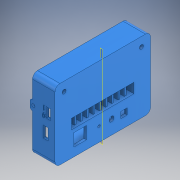
# Autodesk Inventor part: case_front
Saved by Autodesk Inventor 2018 (Build 220112000, 112)
## iProperties
Created: 2018-08-02
Part Number: case_front
Material: Generic
Document SubType Name: Modeling
Designer: Luke
Density: 1 g/cm^3
Appearance: Cyan
Author: Luke
Autodesk Inventor part; units mm, degrees
ref_plane "YZ Plane" through (0, 0, 0) normal (1, 0, 0) x (0, 1, 0)
ref_plane "XZ Plane" through (0, 0, 0) normal (0, 1, 0) x (-1, 0, 0)
sketch "Sketch1" plane through (0, 0, 0) normal (0, 1, 0) x (-1, 0, 0)
  line L0 (0, 0) -> (-76.5, 0)
  line L1 (-76.5, 0) -> (-76.5, 56.5)
  line L2 (-76.5, 56.5) -> (0, 56.5)
  line L3 (0, 56.5) -> (0, 0)
  dimension "d0" = 76.5
  dimension "d1" = 56.5
  constraints: 8 end point, 2 parallel, 1 horizontal, 1 perpendicular
  measures "d0" distance of L0.start L0.end
  measures "d1" distance of L0.end L1.end
extrude "Extrusion1" add sketch "Sketch1" along normal blind 2
ref_plane "Work Plane1" through (76.5, 0, 28.25) normal (0, 0, -1) x (-1, 0, 0)
ref_plane "Work Plane2" through (38.25, 0, 56.5) normal (1, 0, 0) x (0, 0, -1)
sketch "Sketch3" plane through (0, 2, 0) normal (0, 1, 0) x (1, 0, 0)
  line L0 (38.25, 11.3) -> (38.25, -67.8) construction
  line L1 (-15.3, -28.25) -> (91.8, -28.25) construction
  circle A0 centre (7.25, -7.25) radius 1.6
  circle A1 centre (69.25, -7.25) radius 1.6
  circle A2 centre (69.25, -49.25) radius 1.6
  circle A3 centre (7.25, -49.25) radius 1.6
  line L2 (7.25, -7.25) -> (69.25, -7.25) construction
  line L3 (69.25, -7.25) -> (69.25, -49.25) construction
  line L4 (69.25, -49.25) -> (7.25, -49.25) construction
  line L5 (7.25, -49.25) -> (7.25, -7.25) construction
  point P0 (0, 0)
  dimension "d4" = 3.2
  dimension "d5" = 3.2
  dimension "d6" = 3.2
  dimension "d7" = 3.2
  dimension "d8" = 62
  dimension "d9" = 42
  constraints: 8 end point, 4 centre point, 4 coincident, 2 parallel, 1 horizontal, 1 perpendicular, 2 other
  measures "d4" diameter of A0
  measures "d5" diameter of A1
  measures "d6" diameter of A2
  measures "d7" diameter of A3
  measures "d8" distance of L2.start L2.end
  measures "d9" distance of L2.end L3.end
extrude "Extrusion2" cut sketch "Sketch3" against normal up to surface (2 mm away)
sketch "Sketch4" plane through (0, 0, 0) normal (0, -1, 0) x (1, 0, 0)
  line L0 (0, 0) -> (76.5, 0) projected
  line L1 (76.5, 0) -> (76.5, 56.5) projected
  line L2 (76.5, 56.5) -> (0, 56.5) projected
  line L3 (0, 56.5) -> (0, 0) projected
  line L4 (74.5, 2) -> (2, 2)
  line L5 (2, 2) -> (2, 54.5)
  line L6 (2, 54.5) -> (74.5, 54.5)
  line L7 (74.5, 54.5) -> (74.5, 2)
  dimension "d12" = 2
  constraints: 8 end point, 3 other
  measures "d12" distance between parallel lines of L4 L0
extrude "Extrusion3" add sketch "Sketch4" along normal blind 16
sketch "Sketch5" plane through (0, 2, 0) normal (0, 1, 0) x (1, 0, 0)
  circle A0 centre (7.25, -49.25) radius 1.6 construction
  line L0 (15.175, -39.675) -> (25.175, -39.675)
  line L1 (25.175, -39.675) -> (25.175, -49.675)
  line L2 (25.175, -49.675) -> (15.175, -49.675)
  line L3 (15.175, -49.675) -> (15.175, -39.675)
  point P0 (0, 0)
  dimension "d15" = 7.925
  dimension "d16" = 10
  dimension "d17" = 10
  dimension "d18" = 9.575
  constraints: 8 end point, 2 parallel, 1 horizontal, 1 perpendicular
  measures "d15" distance from line of A0.centre L3
  measures "d16" distance of L1.end L2.end
  measures "d17" distance of L0.end L1.end
  measures "d18" distance from line of A0.centre L0
extrude "Extrusion4" cut sketch "Sketch5" against normal up to surface (2 mm away)
sketch "Sketch6" plane through (0, 2, 0) normal (-1, 0, 0) x (0, 0, 1)
  line L0 (17.5, -3.5) -> (25.5, -3.5)
  line L1 (25.5, -3.5) -> (25.5, -7)
  line L2 (25.5, -7) -> (17.5, -7)
  line L3 (17.5, -7) -> (17.5, -3.5)
  line L4 (0, 0) -> (56.5, 0) construction
  line L5 (56.5, 0) -> (56.5, -18) construction
  point P0 (0, -2)
  dimension "d21" = 31
  dimension "d22" = 3.5
  dimension "d23" = 8
  dimension "d24" = 3.5
  constraints: 8 end point, 2 parallel, 1 horizontal, 1 perpendicular
  measures "d21" distance between parallel lines of L5 L1
  measures "d22" distance of L0.end L1.end
  measures "d23" distance of L0.start L0.end
  measures "d24" distance between parallel lines of L0 L4
extrude "Extrusion5" cut sketch "Sketch6" against normal up to surface (2 mm away)
sketch "Sketch7" plane through (0, 2, 0) normal (-1, 0, 0) x (0, 0, 1)
  line L0 (0, 0) -> (56.5, 0) construction
  line L1 (56.5, 0) -> (56.5, -18) construction
  line L2 (31.5, -5.5) -> (40.5, -5.5)
  line L3 (40.5, -5.5) -> (40.5, -9.5)
  line L4 (40.5, -9.5) -> (31.5, -9.5)
  line L5 (31.5, -9.5) -> (31.5, -5.5)
  point P0 (0, -2)
  dimension "d27" = 16
  dimension "d28" = 9
  dimension "d29" = 4
  dimension "d30" = 5.5
  constraints: 8 end point, 2 parallel, 1 horizontal, 1 perpendicular
  measures "d27" distance between parallel lines of L1 L3
  measures "d28" distance of L2.start L2.end
  measures "d29" distance of L4.end L2.start
  measures "d30" distance between parallel lines of L2 L0
extrude "Extrusion6" cut sketch "Sketch7" against normal up to surface (2 mm away)
fillet "Fillet1" radius 4 8 edges at (74.5, -8, 54.5) (76.5, -7, 56.5) (74.5, -8, 2) (76.5, -7, 0) (2, -8, 2) (0, -7, 0) (0, -7, 56.5) (2, -8, 54.5)
sketch "Sketch8" plane through (0, -16, 52.5) normal (-1, 0, 0) x (0, 0, 1)
  line L0 (-52.5, 18) -> (-52.5, 0) construction
  line L1 (0, 0) -> (-48.5, 0) construction
  line L2 (-2, 0) -> (-46.5, 0) projected
  line L3 (-26.5, 0) -> (-34.5, 0)
  line L4 (-34.5, 0) -> (-34.5, -2)
  line L5 (-34.5, -2) -> (-26.5, -2)
  line L6 (-26.5, -2) -> (-26.5, 0)
  line L7 (-30.5, -2) -> (-30.5, 0) construction
  point P0 (-52.5, 16)
  dimension "d34" = 22
  dimension "d35" = 8
  dimension "d36" = 2
  constraints: 10 end point, 2 midpoint, 2 parallel, 1 horizontal, 1 perpendicular, 1 point on line
  measures "d34" distance between parallel lines of L0 L7
  measures "d35" distance of L4.end L5.end
  measures "d36" distance of L3.end L4.end
extrude "Extrusion7" add sketch "Sketch8" against normal up to surface (2 mm away)
sketch "Sketch9" plane through (0, -16, 52.5) normal (-1, 0, 0) x (0, 0, 1)
  line L0 (0, 0) -> (-26.5, 0) construction
  line L1 (-52.5, 18) -> (-52.5, 0) construction
  circle A0 centre (-30.5, 0.75) radius 1.25
  point P0 (-52.5, 16)
  dimension "d39" = 2.5
  dimension "d43" = 0.75
  dimension "d44" = 22
  constraints: 1 centre point
  measures "d39" diameter of A0
  measures "d43" distance from line of A0.centre L0
  measures "d44" distance from line of L1 A0.centre
extrude "Extrusion8" cut sketch "Sketch9" against normal up to surface (2 mm away)
sketch "Sketch10" plane through (0, 2, 0) normal (0, 1, 0) x (1, 0, 0)
  circle A0 centre (7.25, -49.25) radius 1.6 projected
  circle A1 centre (69.25, -49.25) radius 1.6 projected
  line L0 (13.25, -28.75) -> (63.25, -28.75)
  line L1 (63.25, -28.75) -> (63.25, -36.75)
  line L2 (63.25, -36.75) -> (13.25, -36.75)
  line L3 (13.25, -36.75) -> (13.25, -28.75)
  line L4 (7.25, -49.25) -> (69.25, -49.25) construction
  line L5 (38.25, -49.25) -> (38.25, -36.75) construction
  point P0 (0, 0)
  dimension "d45" = 12.5
  dimension "d46" = 8
  dimension "d47" = 50
  constraints: 12 end point, 2 horizontal, 2 midpoint, 2 parallel, 2 perpendicular
  measures "d45" distance from line of L4.start L2
  measures "d46" distance of L2.end L0.start
  measures "d47" distance of L0.start L0.end
extrude "Extrusion9" cut sketch "Sketch10" against normal up to surface (2 mm away) contours L0 L1 L2 L3
sketch "Sketch11" plane through (0, 0, 0) normal (0, -1, 0) x (1, 0, 0)
  line L0 (63.25, 28.75) -> (13.25, 28.75) projected
  line L1 (13.25, 28.75) -> (13.25, 36.75) projected
  line L2 (13.25, 36.75) -> (63.25, 36.75) projected
  line L3 (63.25, 36.75) -> (63.25, 28.75) projected
  line L4 (64.75, 38.25) -> (11.75, 38.25)
  line L5 (11.75, 38.25) -> (11.75, 27.25)
  line L6 (11.75, 27.25) -> (64.75, 27.25)
  line L7 (64.75, 27.25) -> (64.75, 38.25)
  point P0 (0, 0)
  dimension "d50" = 1.5
  constraints: 8 end point, 3 other
  measures "d50" distance between parallel lines of L2 L4
extrude "Extrusion10" add sketch "Sketch11" along normal blind 6
sketch "Sketch12" plane through (0, -6, 0) normal (0, -1, 0) x (1, 0, 0)
  line L0 (13.25, 28.75) -> (13.25, 36.75) projected
  line L1 (13.25, 36.75) -> (63.25, 36.75) projected
  line L2 (63.25, 36.75) -> (63.25, 28.75) projected
  line L3 (63.25, 28.75) -> (13.25, 28.75) projected
  line L4 (64.75, 38.25) -> (11.75, 38.25) projected
  line L5 (11.75, 38.25) -> (11.75, 27.25) projected
  line L6 (11.75, 27.25) -> (64.75, 27.25) projected
  line L7 (64.75, 27.25) -> (64.75, 38.25) projected
  line L8 (63.25, 36.75) -> (13.25, 36.75) construction
  line L9 (38.25, 36.75) -> (38.25, 28.75) construction
  line L10 (37.5, 36.75) -> (37.5, 28.75)
  line L11 (13.25, 28.75) -> (63.25, 28.75) projected
  line L12 (39, 36.75) -> (39, 28.75)
  line L13 (37.5, 36.75) -> (39, 36.75)
  line L14 (37.5, 28.75) -> (39, 28.75)
  point P0 (0, 0)
  dimension "d53" = 1.5
  constraints: 10 end point, 4 point on line, 2 collinear, 2 midpoint, 1 perpendicular, 1 vertical, 1 other
  measures "d53" distance between parallel lines of L12 L10
extrude "Extrusion11" add sketch "Sketch12" against normal blind 6 contours L10 L1 L12 L3
pattern_linear "Rectangular Pattern1" count 9 spacing 5 along (1, 0, 0) of "Extrusion11" first direction both ways yes
sketch "Sketch13" plane through (0, 2, 0) normal (0, 1, 0) x (1, 0, 0)
  circle A0 centre (69.25, -49.25) radius 1.6 construction
  line L0 (52.75, -43.75) -> (57.75, -43.75)
  line L1 (57.75, -43.75) -> (57.75, -48.75)
  line L2 (57.75, -48.75) -> (52.75, -48.75)
  line L3 (52.75, -48.75) -> (52.75, -43.75)
  line L4 (55.25, -43.75) -> (55.25, -48.75) construction
  line L5 (57.75, -46.25) -> (52.75, -46.25) construction
  point P0 (0, 0)
  point P1 (55.25, -46.25)
  dimension "d59" = 14
  dimension "d60" = 3
  dimension "d61" = 5
  dimension "d62" = 5
  constraints: 12 end point, 5 midpoint, 2 parallel, 1 horizontal, 1 perpendicular
  measures "d59" horizontal distance of A0.centre point (55.25, -46.25)
  measures "d60" vertical distance of A0.centre point (55.25, -46.25)
  measures "d61" distance of L2.end L0.start
  measures "d62" distance of L0.start L0.end
extrude "Extrusion12" cut sketch "Sketch13" against normal up to surface (2 mm away)
sketch "Sketch14" plane through (0, 2, 0) normal (0, 1, 0) x (1, 0, 0)
  circle A0 centre (7.25, -49.25) radius 1.6 construction
  circle A1 centre (35.25, -45.25) radius 1
  point P0 (0, 0)
  dimension "d65" = 2
  dimension "d66" = 28
  dimension "d67" = 4
  constraints: 1 centre point
  measures "d65" diameter of A1
  measures "d66" horizontal distance of A1.centre A0.centre
  measures "d67" vertical distance of A0.centre A1.centre
extrude "Extrusion13" cut sketch "Sketch14" against normal up to surface (2 mm away)
sketch "Sketch15" plane through (0, 2, 0) normal (0, 1, 0) x (1, 0, 0)
  circle A0 centre (7.25, -49.25) radius 1.6 construction
  circle A1 centre (45.25, -45.25) radius 2
  point P0 (0, 0)
  dimension "d70" = 38
  dimension "d71" = 4
  dimension "d72" = 4
  constraints: 1 centre point
  measures "d70" horizontal distance of A1.centre A0.centre
  measures "d71" vertical distance of A0.centre A1.centre
  measures "d72" diameter of A1
extrude "Extrusion14" cut sketch "Sketch15" against normal up to surface (2 mm away)
sketch "Sketch16" plane through (0, 2, 0) normal (0, 1, 0) x (1, 0, 0)
  circle A0 centre (45.25, -45.25) radius 2 projected
  circle A1 centre (35.25, -45.25) radius 1 projected
  line L0 (57.75, -43.75) -> (57.75, -48.75) projected
  line L1 (57.75, -48.75) -> (52.75, -48.75) projected
  line L2 (52.75, -48.75) -> (52.75, -43.75) projected
  line L3 (52.75, -43.75) -> (57.75, -43.75) projected
  line L4 (63.25, -28.75) -> (63.25, -36.75) projected
  line L5 (63.25, -36.75) -> (13.25, -36.75) projected
  line L6 (13.25, -36.75) -> (13.25, -28.75) projected
  line L7 (13.25, -28.75) -> (63.25, -28.75) projected
  arc A2 (0, -52.5) -> (4, -56.5) centre (4, -52.5) ccw projected
  line L8 (4, -56.5) -> (72.5, -56.5) projected
  arc A3 (72.5, -56.5) -> (76.5, -52.5) centre (72.5, -52.5) ccw projected
  line L9 (76.5, -52.5) -> (76.5, -4) projected
  arc A4 (76.5, -4) -> (72.5, 0) centre (72.5, -4) ccw projected
  line L10 (72.5, 0) -> (4, 0) projected
  arc A5 (4, 0) -> (0, -4) centre (4, -4) ccw projected
  line L11 (0, -4) -> (0, -52.5) projected
  line L12 (25.175, -39.675) -> (25.175, -49.675) projected
  line L13 (25.175, -49.675) -> (15.175, -49.675) projected
  line L14 (15.175, -49.675) -> (15.175, -39.675) projected
  line L15 (15.175, -39.675) -> (25.175, -39.675) projected
  circle A6 centre (69.25, -49.25) radius 1.6 projected
  circle A7 centre (7.25, -49.25) radius 1.6 projected
  circle A8 centre (69.25, -7.25) radius 1.6 projected
  circle A9 centre (7.25, -7.25) radius 1.6 projected
  point P0 (0, 0)
extrude "Extrusion15" [suppressed]
mirror "Mirror1" about plane through (38.25, 0, 56.5) normal (1, 0, 0) of "Extrusion8", "Extrusion7"
sketch "Sketch17" plane through (0, -16, 52.5) normal (-1, 0, 0) x (0, 0, 1)
  line L0 (-35.21, 8.5792) -> (-35.21, 11.2056) construction
  line L1 (-35.21, 11.2056) -> (-31.6986, 11.2056) construction
  line L2 (-31.6986, 11.2056) -> (-31.6986, 8.5792) construction
  line L3 (-31.6986, 8.5792) -> (-35.21, 8.5792) construction
  line L4 (-29.95, 7.8925) -> (-29.95, 10.5189) construction
  line L5 (-29.95, 10.5189) -> (-26.4386, 10.5189) construction
  line L6 (-26.4386, 10.5189) -> (-26.4386, 7.8925) construction
  line L7 (-26.4386, 7.8925) -> (-29.95, 7.8925) construction
  spline S0 degree 2 poles (-31.9737, 9.5088) (-31.7206, 9.5088) (-31.7206, 9.2557) knots 0 0 0 1 1 1
  spline S1 degree 2 poles (-31.7206, 9.2557) (-31.7206, 9.0027) (-31.9737, 9.0027) knots 0 0 0 1 1 1
  line L8 (-31.9737, 9.0027) -> (-34.9596, 9.0027)
  spline S2 degree 2 poles (-34.9596, 9.0027) (-35.21, 9.0027) (-35.21, 9.2557) knots 0 0 0 1 1 1
  spline S3 degree 2 poles (-35.21, 9.2557) (-35.21, 9.5088) (-34.9596, 9.5088) knots 0 0 0 1 1 1
  line L9 (-34.9596, 9.5088) -> (-31.9737, 9.5088)
  spline S4 degree 2 poles (-28.192, 10.3244) (-27.4941, 10.3244) (-27.0679, 10.0527) knots 0 0 0 1 1 1
  spline S5 degree 2 poles (-27.0679, 10.0527) (-26.4367, 9.741) (-26.4367, 9.2509) knots 0 0 0 1 1 1
  spline S6 degree 2 poles (-26.4367, 9.2509) (-26.4367, 8.7608) (-27.0679, 8.4492) knots 0 0 0 1 1 1
  spline S7 degree 2 poles (-27.0679, 8.4492) (-27.4914, 8.1775) (-28.192, 8.1775) knots 0 0 0 1 1 1
  spline S8 degree 2 poles (-28.192, 8.1775) (-28.8872, 8.1775) (-29.3214, 8.4545) knots 0 0 0 1 1 1
  spline S9 degree 2 poles (-29.3214, 8.4545) (-29.95, 8.7661) (-29.95, 9.2509) knots 0 0 0 1 1 1
  spline S10 degree 2 poles (-29.95, 9.2509) (-29.95, 9.741) (-29.3959, 10.0474) knots 0 0 0 1 1 1
  spline S11 degree 2 poles (-29.3959, 10.0474) (-28.8898, 10.3244) (-28.192, 10.3244) knots 0 0 0 1 1 1
  spline S12 degree 2 poles (-28.1973, 9.8289) (-28.7034, 9.8289) (-29.0603, 9.6744) knots 0 0 0 1 1 1
  spline S13 degree 2 poles (-29.0603, 9.6744) (-29.4359, 9.5146) (-29.4359, 9.2509) knots 0 0 0 1 1 1
  spline S14 degree 2 poles (-29.4359, 9.2509) (-29.4359, 8.9926) (-29.0257, 8.8194) knots 0 0 0 1 1 1
  spline S15 degree 2 poles (-29.0257, 8.8194) (-28.7007, 8.6782) (-28.192, 8.6782) knots 0 0 0 1 1 1
  spline S16 degree 2 poles (-28.192, 8.6782) (-27.6806, 8.6782) (-27.3263, 8.8327) knots 0 0 0 1 1 1
  spline S17 degree 2 poles (-27.3263, 8.8327) (-26.9507, 8.9926) (-26.9507, 9.2509) knots 0 0 0 1 1 1
  spline S18 degree 2 poles (-26.9507, 9.2509) (-26.9507, 9.5093) (-27.3316, 9.6744) knots 0 0 0 1 1 1
  spline S19 degree 2 poles (-27.3316, 9.6744) (-27.6886, 9.8289) (-28.1973, 9.8289) knots 0 0 0 1 1 1
  point P0 (-52.5, 16)
  constraints: 4 other
extrude "Extrusion16" add sketch "Sketch17" along normal blind 0.5
sketch "Sketch18" plane through (4, -16, 56.5) normal (0, 0, 1) x (1, 0, 0)
  line L0 (34.25, 22) -> (34.25, -6) construction
  line L1 (68.5, 0) -> (0, 0) construction
  line L2 (49.25, 0) -> (19.25, 0)
  line L3 (19.25, 0) -> (19.25, 3)
  line L4 (19.25, 3) -> (49.25, 3)
  line L5 (49.25, 3) -> (49.25, 0)
  point P0 (-4, 16)
  dimension "d79" = 3
  dimension "d80" = 30
  constraints: 8 end point, 2 parallel, 1 horizontal, 1 perpendicular, 1 point on line, 1 other
  measures "d79" distance of L2.end L3.end
  measures "d80" distance between parallel lines of L3 L5
extrude "Extrusion17" cut sketch "Sketch18" against normal up to surface (2 mm away)
fillet "Fillet2" radius 2 4 edges at (53.25, -16, 55.5) (53.25, -13, 55.5) (23.25, -16, 55.5) (23.25, -13, 55.5)
sketch "Sketch20" plane through (0, 0, 0) normal (0, -1, 0) x (1, 0, 0)
  circle A0 centre (69.25, 49.25) radius 1.6 projected
  arc A1 (74.5, 50.5) -> (70.5, 54.5) centre (70.5, 50.5) ccw projected
  line L0 (74.5, 50.5) -> (74.5, 26) projected
  line L1 (55.25, 54.5) -> (70.5, 54.5) projected
  line L2 (64.5, 54.5) -> (64.5, 44.5)
  line L3 (64.5, 44.5) -> (74.5, 44.5)
  point P0 (0, 0)
  dimension "d84" = 10
  dimension "d85" = 10
  constraints: 4 end point, 2 point on line, 1 perpendicular, 1 vertical
  measures "d84" distance of L2.end L3.end
  measures "d85" distance of L2.start L2.end
extrude "Extrusion18" add sketch "Sketch20" along normal blind 6.7
sketch "Sketch22" plane through (0, 2, 0) normal (0, 1, 0) x (1, 0, 0)
  circle A0 centre (69.25, -49.25) radius 1.6 projected
  point P0 (0, 0)
extrude "Extrusion19" add sketch "Sketch22" against normal blind 3
mirror "Mirror2" about plane through (38.25, 0, 56.5) normal (1, 0, 0) of "Extrusion18", "Extrusion19"
fillet "Fillet3" radius 2 4 edges at (1, -18, 26) (1, -18, 18) (75.5, -18, 26) (75.5, -18, 18)
equation "\"d5\" = d4"
equation "\"d6\" = d5"
equation "\"d7\" = d6"
body "Solid1"
